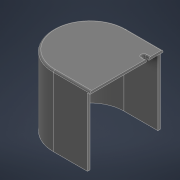
# Autodesk Inventor part: Telo
Saved by Autodesk Inventor 2022 (Build 260153000, 153)
## iProperties
Created: 2021-05-14
Part Number: Telo
Material: Generic
Document SubType Name: Modeling
Designer: jodyn
Density: 1 g/cm^3
Appearance: Gray
Author: jodyn
## iProperties of the stored document Telo_3DPrint.ipt
Created: 2021-05-14
Part Number: Telo_3DPrint
Material: Generic
Document SubType Name: Modeling
Designer: jodyn
Density: 1 g/cm^3
Appearance: Default
Author: jodyn
Autodesk Inventor part; units mm, degrees
ref_plane "YZ Plane" through (0, 0, 0) normal (1, 0, 0) x (0, 1, 0)
ref_plane "XZ Plane" through (0, 0, 0) normal (0, 1, 0) x (-1, 0, 0)
ref_plane "XY Plane" through (0, 0, 0) normal (0, 0, 1) x (1, 0, 0)
sketch "Sketch1" plane through (0, 0, 0) normal (0, 1, 0) x (-1, 0, 0)
  line L0 (0, 40) -> (-35, 40)
  line L1 (-35, -40) -> (0, -40)
  arc A0 (0, -40) -> (0, 40) centre (0, 0) ccw
  line L2 (-35, 43) -> (0, 43)
  arc A1 (0, -43) -> (0, 43) centre (0, 0) ccw
  line L3 (0, -43) -> (-35, -43)
  line L4 (-35, 43) -> (-40, 43)
  line L5 (-40, 43) -> (-40, 40)
  line L6 (-40, 40) -> (-35, 40)
  line L7 (-35, -40) -> (-40, -40)
  line L8 (-40, -40) -> (-40, -43)
  line L9 (-40, -43) -> (-35, -43)
  dimension "d7" = 3
  constraints: 20 end point, 4 parallel, 4 point on circle, 2 centre point, 2 horizontal, 2 perpendicular, 2 other
  measures "d7" radial gap between concentric circles of A0 A1
extrude "Extrusion1" add sketch "Sketch1" along normal blind 80
sketch "Sketch2" plane through (0, 80, 0) normal (0, 1, 0) x (1, 0, 0)
  line L0 (40, 43) -> (0, 43) projected
  arc A0 (0, 43) -> (0, -43) centre (0, 0) ccw projected
  line L1 (0, -43) -> (40, -43) projected
  line L2 (40, -43) -> (43, -43)
  line L3 (43, -43) -> (43, -40)
  line L4 (0, 40) -> (40, 40) projected
  line L5 (43, 40) -> (43, 43)
  line L6 (43, 43) -> (40, 43)
  line L7 (43, -40) -> (43, 40)
  constraints: 10 end point, 1 horizontal, 1 perpendicular, 1 vertical
extrude "Extrusion2" add sketch "Sketch2" along normal blind 3
sketch "Sketch3" plane through (0, 83, 0) normal (0, 1, 0) x (1, 0, 0)
  line L0 (43, -43) -> (43, 43) projected
  line L1 (43, 23.4737) -> (38.5, 23.4737)
  line L2 (38.5, 26.4737) -> (43, 26.4737)
  line L3 (43, 26.4737) -> (43, 23.4737)
  arc A0 (38.5, 26.4737) -> (38.5, 23.4737) centre (38.5, 24.9737) ccw
  constraints: 6 end point, 2 point on circle, 2 tangent, 1 centre point, 1 horizontal, 1 parallel, 1 point on line
extrude "Extrusion3" cut sketch "Sketch3" against normal blind 3
fillet "Fillet1" radius 2 6 edges at (21.5, 83, 43) (21.5, 83, -43) (-43, 83, 0) (37, 83, -24.9737) (40.75, 83, -26.4737) (40.75, 83, -23.4737)
body "Solid1"
